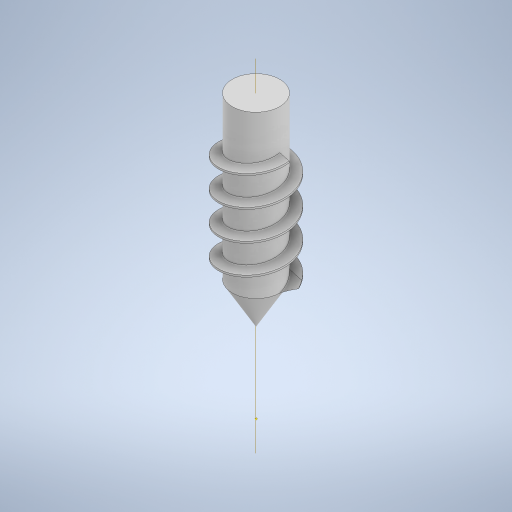
# Autodesk Inventor part: TipNr8
Saved by Autodesk Inventor 2023.2 (Build 272271030, 271C)
## iProperties
Created: 2022-11-02
Part Number: TipNr8
Material: Generisch
Document SubType Name: Modeling
Designer: mehan
Density: 1 g/cm^3
Appearance: Vorgabe
Author: mehan
Autodesk Inventor part; units mm, degrees
ref_plane "YZ Plane" through (0, 0, 0) normal (1, 0, 0) x (0, 1, 0)
ref_plane "XZ Plane" through (0, 0, 0) normal (0, 1, 0) x (-1, 0, 0)
ref_plane "XY Plane" through (0, 0, 0) normal (0, 0, 1) x (1, 0, 0)
sketch "Skizze1" plane through (0, 0, 0) normal (0, 0, 1) x (1, 0, 0)
  line L0 (0, -70) -> (40.4145, 0)
  line L1 (40.4145, 0) -> (40.4145, 215)
  line L2 (40.4145, 215) -> (0, 215)
  line L3 (0, 215) -> (0, -70)
  point P0 (0, 0)
  dimension "d0" = 70
  dimension "d2" = 215
  dimension "d33" = 40.4145
  dimension "d34" = 30
  constraints: 8 end point, 2 vertical, 1 perpendicular
  measures "d0" distance of point (0, 0) L0.start
  measures "d2" distance of L0.end L1.end
  measures "d33" distance of L1.end L2.end
  measures "d34" angle of L0 L3
sketch "Skizze2" plane through (0, 0, 0) normal (0, 0, 1) x (1, 0, 0)
  line L0 (0, -70) -> (40.4145, 0) projected
  line L1 (40.4145, 0) -> (40.4145, 150) projected
  line L2 (40.4145, 9.2376) -> (40.4145, 0)
  line L3 (40.4145, 0) -> (56.4145, 0)
  line L4 (56.4145, 0) -> (56.4145, 3)
  line L5 (56.4145, 3) -> (40.4145, 6.9892)
  point P0 (0, 0)
  dimension "d22" = 16
  dimension "d23" = 3
  dimension "d35" = 104
  dimension "d36" = 3.9893
  constraints: 8 end point, 2 point on line, 1 collinear, 1 horizontal, 1 perpendicular
  measures "d22" distance of L1.start L3.end
  measures "d23" distance of L3.end L4.end
  measures "d35" angle of L4 L5
  measures "d36" vertical distance of L4.end L5.end
coil "Spirale1" sketch "Skizze2" operation add axis through (0, -10, 0) along (0, 1, 0) pitch 50 turns 4 hand right
revolve "Umdrehung1" add sketch "Skizze1" angle 360 about axis through (0, 215, 0) along (0, -1, 0)
chamfer "Fase4" distance 6.7 distance2 30 1 edges at (48.4145, 4.9946, 0) measured on face at (48.2936, 4.5095, 0)
sketch "Skizze3" plane through (0, 0, 0) normal (0, 0, 1) x (1, 0, 0)
  point P0 (0, 0)
sketch "Skizze4" plane through (0, 0, 0) normal (0, 0, 1) x (1, 0, 0)
  line L0 (-40.4145, 215) -> (40.4145, 215) projected
  line L1 (0, 215) -> (0, 275)
  line L2 (0, 275) -> (40.4145, 275)
  line L3 (40.4145, 275) -> (40.4145, 215)
  line L4 (0, 215) -> (40.4145, 215)
  line L5 (0, -55) -> (0, 330) projected
  point P0 (0, 0)
  dimension "d41" = 60
  constraints: 8 end point, 3 perpendicular, 1 midpoint, 1 vertical
  measures "d41" distance of L1.start L1.end
revolve "Umdrehung2" add sketch "Skizze4" angle 360 about axis through (0, -10, 0) along (0, 1, 0)
scale "Skalierung1" factors (0.4, 0.4, 0.4) then translate (0, 82.5, 0) bodies 1
